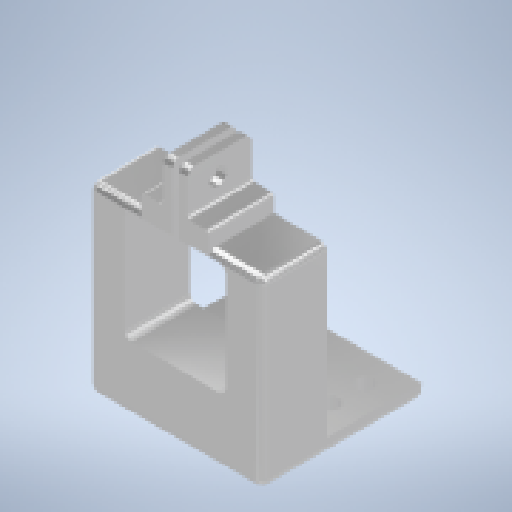
# Autodesk Inventor part: Bracket
Saved by Autodesk Inventor 2025.3 (Build 293356000, 356)
## iProperties
Created: 2009-08-20
Part Number: Bracket
Material: Aluminum 6061
Document SubType Name: Modeling
Designer: Haggag
Density: 2.7 g/cm^3
Appearance: Aluminum - Flat
Author: Haggag
Autodesk Inventor part; units mm, degrees
ref_plane "YZ Plane" through (0, 0, 0) normal (1, 0, 0) x (0, 1, 0)
ref_plane "XZ Plane" through (0, 0, 0) normal (0, 1, 0) x (-1, 0, 0)
ref_plane "XY Plane" through (0, 0, 0) normal (0, 0, 1) x (1, 0, 0)
sketch "Sketch3" plane through (0, 0, 0) normal (0, 0, 1) x (1, 0, 0)
  line L0 (9.100633, 7.96547) -> (9.089027, 7.96547)
  line L1 (7.193736, 11.000646) -> (7.193757, 12.332986)
  line L2 (10.100661, 11.015006) -> (10.101877, 12.347346)
  line L3 (8.205862, 7.96547) -> (8.205862, 12.332986)
  line L4 (9.100633, 12.345156) -> (9.100633, 7.96547)
  line L5 (4.504617, 7.150409) -> (4.504617, 8.767837)
  line L6 (12.776796, 8.767837) -> (12.776796, 7.150409)
  line L7 (7.193757, 12.332986) -> (7.193757, 14.390131)
  line L8 (7.193757, 14.390131) -> (8.205862, 14.390131)
  line L9 (8.205862, 14.390131) -> (8.205862, 12.332986)
  line L10 (9.100633, 12.345156) -> (9.100633, 14.390131)
  line L11 (10.101877, 12.347346) -> (10.101877, 14.390131)
  line L12 (10.101877, 14.390131) -> (9.100633, 14.390131)
  line L13 (19.293553, 6.283983) -> (19.293553, -8.230127)
  line L14 (18.427127, -15.238701) -> (-1.145933, -15.238701)
  line L15 (-2.012359, -8.230259) -> (-2.012359, 6.283983)
  line L16 (4.504617, 7.150409) -> (-1.145933, 7.150409)
  line L17 (12.776796, 7.150409) -> (18.427127, 7.150409)
  arc A0 (-1.145933, 7.150409) -> (-2.012359, 6.283983) centre (-1.145933, 6.283983) ccw
  arc A1 (19.293553, 6.283983) -> (18.427127, 7.150409) centre (18.427127, 6.283983) ccw
  line L18 (-1.145933, -15.238701) -> (-2.012359, -15.238701)
  line L19 (-2.012359, -15.238701) -> (-2.012359, -8.230259)
  line L20 (18.427127, -15.238701) -> (19.293553, -15.238701)
  line L21 (19.293553, -15.238701) -> (19.293553, -8.230127)
  line L22 (9.100633, -7.254895) -> (9.089027, -7.254895)
  line L23 (6.288137, -7.254895) -> (8.205862, -7.254895)
  line L24 (9.100633, -7.254895) -> (10.99283, -7.255376)
  line L25 (8.205862, 7.96547) -> (8.205862, 7.150409)
  line L26 (9.100633, 7.96547) -> (9.100633, 7.150637)
  line L27 (8.205862, -7.254895) -> (9.100633, -7.254895)
  line L28 (8.205862, 7.150409) -> (8.205862, 6.530192)
  line L29 (9.100633, 7.150637) -> (9.100633, 6.528785)
  line L30 (3.31641, -7.254895) -> (13.964785, -7.254895)
  line L31 (14.830785, -6.388895) -> (14.830785, 5.664192)
  line L32 (2.45041, 5.664192) -> (2.45041, -6.388895)
  arc A2 (2.45041, -6.388895) -> (3.31641, -7.254895) centre (3.31641, -6.388895) ccw
  arc A3 (13.964785, -7.254895) -> (14.830785, -6.388895) centre (13.964785, -6.388895) ccw
  arc A4 (3.31641, 6.530192) -> (2.45041, 5.664192) centre (3.31641, 5.664192) ccw
  arc A5 (14.830785, 5.664192) -> (13.964785, 6.530192) centre (13.964785, 5.664192) ccw
  line L33 (13.964785, 6.530192) -> (9.100633, 6.530192)
  line L34 (8.205862, 6.530192) -> (3.31641, 6.530192)
  line L35 (5.004617, 9.267837) -> (6.693736, 9.267837)
  line L36 (12.100661, 9.267837) -> (12.276796, 9.267837)
  line L37 (10.100661, 11.015006) -> (10.100661, 11.267837)
  line L38 (7.193736, 11.000646) -> (7.193736, 9.767837)
  arc A6 (6.693736, 9.267837) -> (7.193736, 9.767837) centre (6.693736, 9.767837) ccw
  line L39 (12.100661, 9.267837) -> (10.600661, 9.267837)
  line L40 (10.100661, 9.767837) -> (10.100661, 11.015006)
  arc A7 (10.100661, 9.767837) -> (10.600661, 9.267837) centre (10.600661, 9.767837) ccw
  arc A8 (12.776796, 8.767837) -> (12.276796, 9.267837) centre (12.276796, 8.767837) ccw
  arc A9 (5.004617, 9.267837) -> (4.504617, 8.767837) centre (5.004617, 8.767837) ccw
  point P0 (4.504617, 9.267837)
  point P1 (12.776796, 9.267837)
  dimension "d37" = 0.866
  dimension "d38" = 12.05309
  dimension "d52" = 0.5
  dimension "d53" = 0.5
  dimension "d54" = 0.5
  constraints: 82 end point, 22 tangent, 20 point on circle, 13 perpendicular, 10 centre point, 7 point on line, 7 vertical, 6 parallel, 5 equal radius, 5 horizontal
  measures "d37" radius of A2
  measures "d38" distance of L32.start L32.end
  measures "d52" radius of A6
  measures "d53" radius of A7
  measures "d54" radius of A8
extrude "Extrusion2" add sketch "Sketch3" along normal blind 8
sketch "Sketch5" plane through (-13.168282, -15.238701, 0) normal (0, -1, 0) x (1, 0, 0)
  line L0 (11.155547, 0) -> (32.464412, 0)
  line L1 (32.464412, 0) -> (32.464412, -11.858092)
  line L2 (32.464412, -11.858092) -> (11.155547, -11.858092)
  line L3 (11.155547, -11.858092) -> (11.155547, 0)
  point P0 (13.168282, 0)
  constraints: 8 end point, 2 parallel, 1 horizontal, 1 perpendicular
extrude "Extrusion4" add sketch "Sketch5" against normal blind 1.84
fillet "Fillet1" radius 1 2 edges at (-2.0124, -15.2387, 4) (19.2936, -15.2387, 4)
fillet "Fillet2" radius 1 9 edges at (19.0007, -14.9458, 8) (19.2936, -3.9774, 8) (19.0398, 6.8966, 8) (15.602, 7.1504, 8) (-1.7195, -14.9458, 8) (-2.0124, -3.9774, 8) (-1.7586, 6.8966, 8) (1.6793, 7.1504, 8) (8.6406, -15.2387, 8)
sketch "Sketch6" plane through (-13.168282, -13.398701, 0) normal (0, 1, 0) x (1, 0, 0)
  line L0 (45.181147, 9.319827) -> (47.181147, 9.319827)
  line L1 (32.464412, 0) -> (32.464412, 11.858092)
  line L2 (-1.835688, 0) -> (-1.835688, 9.319827)
  line L3 (11.155547, 11.858092) -> (32.464412, 11.858092)
  line L4 (21.587059, 0) -> (8.300574, 0)
  circle A0 centre (14.570473, 3.844832) radius 1.05
  line L5 (21.80998, 11.858092) -> (21.80998, 0.522822)
  line L6 (32.464412, 5.929046) -> (11.155547, 5.929046)
  line L7 (11.155547, 11.858092) -> (11.155547, 0)
  circle A1 centre (29.049486, 3.844832) radius 1.05
  circle A2 centre (14.570473, 8.01326) radius 1.05
  circle A3 centre (29.049486, 8.01326) radius 1.05
  point P0 (13.168282, 0)
  point P1 (47.181147, 0)
  point P2 (0, 9.319827)
  point P3 (30.020574, 0)
  point P4 (15.160574, 0)
  dimension "d50" = 2.1
  constraints: 4 centre point, 4 end point, 3 symmetric about line, 1 midpoint, 1 vertical, 7 other
  measures "d50" diameter of A1
extrude "Extrusion5" cut sketch "Sketch6" against normal blind 3.2 contours A0 | A1 | A2 | A3
fillet "Fillet3" radius 1 4 edges at (9.6013, 14.3901, 8) (9.6013, 14.3901, 0) (7.6998, 14.3901, 8) (7.6998, 14.3901, 0)
fillet "Fillet4" radius 1 2 edges at (-2.0127, -15.2387, -5.929) (19.2961, -15.2387, -5.929)
sketch "Sketch7" plane through (7.193746, 11.000646, 0) normal (-1, 0.0000083, 0) x (0, 0, 1)
  point P0 (0, -11.000705)
  point P1 (4.229329, 0.867734)
hole "Hole1" at (7.193754, 11.86838, 4.229329) direction (1, -0.0000083, 0) diameter 2.1 end through all
fillet "Fillet5" radius 0.5 6 edges at (8.6417, -13.3987, -11.8581) (19.0032, -14.9458, -11.8581) (19.2961, -13.8187, -11.8581) (-1.7198, -14.9458, -11.8581) (-2.0127, -13.8187, -11.8581) (8.6417, -15.2387, -11.8581)
body "Solid3"
